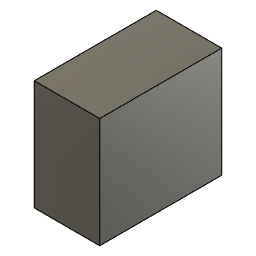
ESC (Autodesk Fusion 360 design; units mm, degrees)
Autodesk Fusion 360 part; units mm, degrees
sketch "Sketch1" plane through (0, 0, 0) normal (0, 1, 0) x (1, 0, 0)
  line L0 (-11, 20.5) -> (11, 20.5)
  line L1 (11, 20.5) -> (11, -20.5)
  line L2 (11, -20.5) -> (-11, -20.5)
  line L3 (-11, -20.5) -> (-11, 20.5)
  line L4 (-11, 20.5) -> (11, -20.5) construction
  line L5 (11, 20.5) -> (-11, -20.5) construction
  dimension "d1" = 41
  dimension "d2" = 22
  constraint perpendicular L0 L1
  constraint parallel L0 L2
  constraint parallel L1 L3
  constraint horizontal L0
  constraint coincident L4 origin
  constraint coincident L5 origin
  measures "d1" distance of L0.end L1.end
  measures "d2" distance of L1.end L2.end
extrude "Extrude1" add sketch "Sketch1" along normal blind 37
